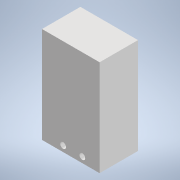
# Autodesk Inventor part: 汽缸
Saved by Autodesk Inventor 2020 (Build 240168000, 168)
## iProperties
Created: 2023-03-07
Part Number: 汽缸
Material: 一般
Document SubType Name: Modeling
Designer: robot
Density: 1 g/cm^3
Appearance: 預設
Author: robot
Autodesk Inventor part; units mm, degrees
ref_plane "YZ Plane" through (0, 0, 0) normal (1, 0, 0) x (0, 1, 0)
ref_plane "XZ Plane" through (0, 0, 0) normal (0, 1, 0) x (-1, 0, 0)
ref_plane "XY Plane" through (0, 0, 0) normal (0, 0, 1) x (1, 0, 0)
sketch "草圖1" plane through (0, 0, 0) normal (0, 0, 1) x (1, 0, 0)
  line L0 (50, 0) -> (50, 100)
  line L1 (50, 100) -> (0, 100)
  line L2 (0, 100) -> (0, 0)
  line L3 (50, 0) -> (33, 0)
  line L4 (33, 0) -> (24.5, 0)
  circle A0 centre (17, 3) radius 1.5
  circle A1 centre (35, 3) radius 1.5
  line L5 (0, 0) -> (50, 0)
  dimension "d0" = 50
  dimension "d4" = 3
  dimension "d5" = 100
  dimension "d7" = 3
  dimension "d22" = 18
  dimension "d23" = 3
  dimension "d24" = 15
  constraints: 12 end point, 2 centre point, 2 horizontal, 1 parallel
  measures "d0" distance of L2.end L0.start
  measures "d4" diameter of A0
  measures "d5" distance of L1.end L2.end
  measures "d7" diameter of A1
  measures "d22" distance between centres of A0 A1
  measures "d23" distance from line of L5 A0.centre
  measures "d24" distance from line of L0 A1.centre
extrude "擠出1" add sketch "草圖1" along normal blind 20
sketch "草圖2" plane through (0, 0, 0) normal (0, -1, 0) x (1, 0, 0)
  line L0 (0, 20) -> (50, 20) projected
  line L1 (0, 0) -> (50, 0) projected
  line L2 (0, 0) -> (0, 20) projected
  line L3 (50, 0) -> (50, 20) projected
  line L4 (50, 5) -> (0, 5)
  line L5 (0, 5) -> (0, 15)
  line L6 (0, 15) -> (50, 15)
  line L7 (50, 15) -> (50, 5)
  point P0 (15, 22.5)
  point P1 (0, 5)
  dimension "d13" = 0
  dimension "d14" = 0
  dimension "d15" = 5
  dimension "d16" = 10
  constraints: 8 end point, 2 parallel, 1 horizontal, 1 perpendicular
  measures "d13" distance between parallel lines of L3 L7
  measures "d14" distance between parallel lines of L2 L5
  measures "d15" distance between parallel lines of L0 L6
  measures "d16" distance between parallel lines of L4 L6
extrude "擠出2" cut sketch "草圖2" against normal blind 20 contours L6 L3 L4 L2
sketch "草圖3" plane through (0, 0, 0) normal (0, 0, -1) x (-1, 0, 0)
  circle A0 centre (-25, 80) radius 10
  line L0 (-50, 100) -> (0, 100) projected
  line L1 (0, 100) -> (0, 0) projected
  circle A1 centre (-8.821, 80) radius 2.067
  circle A2 centre (-41.179, 80) radius 2.067
  line L2 (-25, 80) -> (-8.821, 80)
  line L3 (-25, 80) -> (-41.179, 80)
  dimension "d17" = 20
  dimension "d18" = 20
  dimension "d19" = 25
  dimension "d27" = 4.134
  dimension "d29" = 4.134
  dimension "d30" = 16.179
  dimension "d31" = 16.179
  dimension "d32" = 0
  dimension "d33" = 0
  dimension "d34" = 0
  dimension "d35" = 0
  constraints: 4 end point, 3 centre point, 2 horizontal
  measures "d17" diameter of A0
  measures "d18" distance from line of L0 L2.start
  measures "d19" distance from line of L1 L2.start
  measures "d27" diameter of A1
  measures "d29" diameter of A2
  measures "d30" distance of L2.start L3.end
  measures "d31" distance of L2.start L2.end
  measures "d32" distance of L2.end A1.centre
  measures "d33" distance of L2.end A1.centre
  measures "d34" distance of L3.end A2.centre
  measures "d35" distance of L3.end A2.centre
extrude "擠出3" cut sketch "草圖3" against normal blind 20
